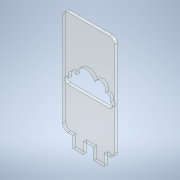
# Autodesk Inventor part: Scheibe
Saved by Autodesk Inventor 2021 (Build 250183000, 183)
## iProperties
Created: 2021-03-05
Part Number: Scheibe
Material: Glas
Document SubType Name: Modeling
Designer: Tilman
Density: 2.18 g/cm^3
Appearance: Klar
Author: Tilman
Autodesk Inventor part; units mm, degrees
ref_plane "YZ Plane" through (0, 0, 0) normal (1, 0, 0) x (0, 1, 0)
ref_plane "XZ Plane" through (0, 0, 0) normal (0, 1, 0) x (-1, 0, 0)
ref_plane "XY Plane" through (0, 0, 0) normal (0, 0, 1) x (1, 0, 0)
sketch "Skizze1" plane through (0, 0, 0) normal (0, 0, 1) x (1, 0, 0)
  line L0 (0, 5) -> (0, 95)
  line L1 (5, 100) -> (45, 100)
  line L2 (50, 95) -> (50, 5)
  arc A0 (5, 100) -> (0, 95) centre (5, 95) ccw
  arc A1 (50, 95) -> (45, 100) centre (45, 95) ccw
  arc A2 (45, 0) -> (50, 5) centre (45, 5) ccw
  arc A3 (0, 5) -> (5, 0) centre (5, 5) ccw
  line L3 (10, 0) -> (10, -11)
  line L4 (10, -11) -> (20, -11)
  line L5 (20, -11) -> (20, 0)
  line L6 (30, 0) -> (30, -11)
  line L7 (30, -11) -> (40, -11)
  line L8 (40, -11) -> (40, 0)
  line L9 (5, 0) -> (10, 0)
  line L10 (20, 0) -> (30, 0)
  line L11 (40, 0) -> (45, 0)
  line L12 (5, 40) -> (45, 40)
  arc A4 (6.0261, 45.8191) -> (5, 40) centre (5, 43) ccw
  arc A5 (45, 40) -> (46.0261, 45.8191) centre (45, 43) ccw
  arc A6 (46.0261, 45.8191) -> (41.3553, 51.3855) centre (42.4089, 47.5268) ccw
  arc A7 (13.45, 52.0485) -> (6.0261, 45.8191) centre (10.5305, 47.9894) ccw
  arc A8 (31.0213, 55.1468) -> (13.45, 52.0485) centre (22.442, 52.4271) ccw
  line L13 (5, 40) -> (6.0261, 45.8191) construction
  line L14 (6.0261, 45.8191) -> (13.45, 52.0485) construction
  line L15 (13.45, 52.0485) -> (31.0213, 55.1468) construction
  line L16 (41.3553, 51.3855) -> (46.0261, 45.8191) construction
  line L17 (45, 40) -> (46.0261, 45.8191) construction
  arc A9 (41.3553, 51.3855) -> (31.0213, 55.1468) centre (36.2306, 53.3825) ccw
  line L18 (31.0213, 55.1468) -> (41.3553, 51.3855) construction
  point P0 (0, 0)
  point P1 (25, 40)
  point P2 (25, 0)
  dimension "d1" = 50
  dimension "d3" = 5
  dimension "d4" = 11
  dimension "d5" = 10
  dimension "d6" = 100
  dimension "d15" = 40
  dimension "d24" = 40
  dimension "d28" = 3
  dimension "d29" = 3
  dimension "d30" = 100
  dimension "d31" = 4
  dimension "d32" = 130
  dimension "d33" = 80
  dimension "d34" = 140
  dimension "d35" = 5
  dimension "d36" = 9
  dimension "d37" = 5.5
  dimension "d38" = 150
  dimension "d39" = 150
  dimension "d40" = 12.0485
  dimension "d41" = 11.3855
  constraints: 38 end point, 20 point on circle, 10 centre point, 9 tangent, 6 horizontal, 5 equal length, 3 equal radius, 3 horizontal alignment, 3 vertical, 2 midpoint, 2 parallel, 2 vertical alignment, 1 perpendicular
  measures "d1" distance between parallel lines of L2 L0
  measures "d3" radius of A0
  measures "d4" distance of L3.start L3.end
  measures "d5" distance of L3.end L4.end
  measures "d6" distance between parallel lines of L10 L1
  measures "d15" distance of L12.start L12.end
  measures "d24" distance between parallel lines of L10 L12
  measures "d28" radius of A4
  measures "d29" radius of A5
  measures "d30" angle of L12 L17
  measures "d31" radius of A6
  measures "d32" angle of L17 L16
  measures "d33" angle of L12 L13
  measures "d34" angle of L13 L14
  measures "d35" radius of A7
  measures "d36" radius of A8
  measures "d37" radius of A9
  measures "d38" angle of L15 L14
  measures "d39" angle of L16 L18
  measures "d40" distance from line of L12 L14.end
  measures "d41" distance from line of L12 L16.start
extrude "Extrusion1" add sketch "Skizze1" along normal blind 3
